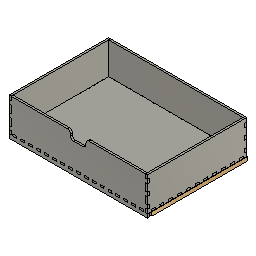
drawer (Autodesk Fusion 360 design; units mm, degrees)
Autodesk Fusion 360 part; units mm, degrees
sketch "Drawer base geometry" plane through (0, 0, 0) normal (0, 0, 1) x (1, 0, 0)
  line L0 (0, 0) -> (362, 0)
  line L1 (362, 0) -> (362, 260)
  line L2 (362, 260) -> (0, 260)
  line L3 (0, 260) -> (0, 0)
  line L4 (1, 0) -> (361, 0)
  line L5 (361, 0) -> (361, 259)
  line L6 (361, 259) -> (1, 259)
  line L7 (1, 259) -> (1, 0)
  line L8 (6, 5) -> (356, 5)
  line L9 (356, 5) -> (356, 254)
  line L10 (356, 254) -> (6, 254)
  line L11 (6, 254) -> (6, 5)
  point P0 (1, 259)
  dimension "d14" = 362
  dimension "d15" = 260
  dimension "d16" = 1
  dimension "d17" = 1
  dimension "d18" = 1
  dimension "d21" = 5
  dimension "d22" = 5
  dimension "d23" = 5
  dimension "d24" = 5
  constraint horizontal L0
  constraint vertical L1
  constraint horizontal L2
  constraint vertical L3
  constraint coincident L0.start L3.end
  constraint horizontal L4
  constraint vertical L5
  constraint horizontal L6
  constraint vertical L7
  constraint horizontal L8
  constraint vertical L9
  constraint horizontal L10
  constraint vertical L11
  constraint collinear L0 L4
  constraint coincident P0 L6.end
  measures "d14" distance of L0.start L0.end
  measures "d15" distance of L0.start L2.end
  measures "d16" distance of L3 L7
  measures "d17" distance of L1 L5
  measures "d18" distance of L2 L6
  measures "d21" distance of L6 L10
  measures "d22" distance of L0 L8
  measures "d23" distance of L5 L9
  measures "d24" distance of L7 L11
ref_plane "WorkPlane1" through (6, 129.5, 0) normal (-1, 0, 0) x (0, -1, 0)
ref_plane "WorkPlane2" through (181, 254, 0) normal (0, 1, 0) x (-1, 0, 0)
sketch "Tabs side" plane through (6, 99.5, 0) normal (-1, 0, 0) x (0, 1, 0)
  line L0 (-99.5, 0) -> (159.5, 0)
  line L1 (159.5, 0) -> (159.5, -88)
  line L2 (159.5, -88) -> (-99.5, -88)
  line L3 (-99.5, -88) -> (-99.5, 0)
  line L4 (-89.5, -5) -> (-79.5, -5)
  line L5 (-79.5, -5) -> (-79.5, 0)
  line L6 (-79.5, 0) -> (-89.5, 0)
  line L7 (-89.5, 0) -> (-89.5, -5)
  line L8 (-99.5, -44) -> (159.5, -44) construction
  line L9 (30, -88) -> (30, 0) construction
  line L10 (-99.5, -10) -> (-94.5, -10)
  line L11 (-94.5, -10) -> (-94.5, -20)
  line L12 (-94.5, -20) -> (-99.5, -20)
  line L13 (-99.5, -20) -> (-99.5, -10)
  point P0 (-99.5, 0)
  dimension "d27" = 259
  dimension "d28" = 88
  dimension "d36" = 10
  dimension "d37" = 10
  dimension "d38" = 5
  dimension "d39" = 10
  dimension "d40" = 5
  dimension "d41" = 10
  constraint horizontal L0
  constraint vertical L1
  constraint horizontal L2
  constraint vertical L3
  constraint coincident P0 L0.start
  constraint horizontal L4
  constraint vertical L5
  constraint horizontal L6
  constraint vertical L7
  constraint midpoint L3 L8.start
  constraint midpoint L1 L8.end
  constraint midpoint L2 L9.start
  constraint coincident L0 L9.end
  constraint perpendicular L0 L9
  constraint collinear L0 L6
  constraint horizontal L10
  constraint vertical L11
  constraint horizontal L12
  constraint vertical L13
  constraint collinear L3 L13
  measures "d27" distance of L1.end L2.end
  measures "d28" distance of P0 L2.end
  measures "d36" distance of L3 L7
  measures "d37" distance of L4.start L4.end
  measures "d38" distance of L0 L4
  measures "d39" distance of L0 L10
  measures "d40" distance of L3 L11
  measures "d41" distance of L10 L12
extrude "Extrude1" add sketch "Tabs side" along normal blind 5 contours L0 L1 L2 L3 L4 L5 L7 L10 L11 L12 makes body 1
ref_plane "WorkPlane3" through (3.5, 139.5, 44) normal (0, 0, -1) x (0, -1, 0)
ref_plane "WorkPlane4" through (3.5, 129.5, 54) normal (0, -1, 0) x (0, 0, 1)
mirror "Mirror2" about plane through (3.5, 129.5, 54) normal (0, -1, 0) of 3 faces at (4.3333, 5, 13.3333) (4.3333, 3.3333, 20) (4.3333, 1.6667, 10) on bodies 1
pattern_linear "R-Pattern2" count 3 spacing 29 along (0, 0, 1) of 6 faces at (4.3333, 5, 13.3333) (4.3333, 3.3333, 20) (4.3333, 1.6667, 10) (4.3333, 257.3333, 10) (4.3333, 254, 13.3333) (4.3333, 255.6667, 20) on bodies 1
pattern_linear "R-Pattern3" count 11 spacing 22.9 along (0, 1, 0) of 3 faces at (4.3333, 10, 1.6667) (4.3333, 13.3333, 5) (4.3333, 20, 3.3333) on bodies 1
sketch "Tab rear" plane through (125, 254, 0) normal (0, 1, 0) x (1, 0, 0)
  line L0 (-124, -88) -> (-124, 0)
  line L1 (-114, 0) -> (-104, 0)
  line L2 (-104, 0) -> (-104, -5)
  line L3 (-104, -5) -> (-114, -5)
  line L4 (-114, -5) -> (-114, 0)
  line L5 (-124, 0) -> (236, 0)
  line L6 (236, 0) -> (236, -88)
  line L7 (236, -88) -> (-124, -88)
  point P0 (-124, 0)
  dimension "d61" = 10
  dimension "d63" = 10
  dimension "d100" = 360
  dimension "d101" = 88
  dimension "d102" = 5
  constraint vertical L0
  constraint coincident P0 L0.end
  constraint horizontal L1
  constraint vertical L2
  constraint horizontal L3
  constraint vertical L4
  constraint perpendicular L4 L5
  constraint perpendicular L5 L6
  constraint parallel L5 L7
  constraint collinear L1 L5
  measures "d61" distance of L0 L4
  measures "d63" distance of L2 L4
  measures "d100" distance of P0 L5.end
  measures "d101" distance of L5 L7
  measures "d102" distance of L3 L5
extrude "Extrude2" add sketch "Tab rear" along normal blind 5 separate body contours L0 L2 L3 L4 L5 L6 L7 makes body 2
pattern_linear "R-Pattern4" count 17 spacing 20.625 along (1, 0, 0) of 3 faces at (11, 255.6667, 3.3333) (17.6667, 255.6667, 5) (21, 255.6667, 1.6667) on bodies 2
ref_plane "WorkPlane5" through (181, 0, 0) normal (1, 0, 0) x (0, 1, 0)
mirror "Mirror3" about plane through (181, 0, 0) normal (1, 0, 0) of bodies 1 makes body 3
combine "Combine1" operation cut target body 2 tool bodies 1 3 keep tools
ref_plane "WorkPlane6" through (0, 129.5, 0) normal (0, 1, 0) x (0, 0, 1)
mirror "Mirror4" about plane through (0, 129.5, 0) normal (0, 1, 0) of bodies 2 makes body 4
extrude "Extrude3" add sketch "Drawer base geometry" along normal blind 5 separate body contours L0 L4 L5 L6 L7 | L8 L9 L10 L11 makes body 5
combine "Combine2" operation cut target body 5 tool bodies 2 1 3 4 keep tools
sketch "Front lip" plane through (0, 0, 0) normal (0, 1, 0) x (1, 0, 0)
  line L0 (1, 0) -> (361, 0)
  line L1 (361, 0) -> (361, 9.5)
  line L2 (361, 9.5) -> (1, 9.5)
  line L3 (1, 9.5) -> (1, 0)
  point P0 (1, 0)
  dimension "d78" = 360
  dimension "d80" = 9.5
  constraint horizontal L0
  constraint vertical L1
  constraint horizontal L2
  constraint vertical L3
  constraint coincident P0 L0.start
  measures "d78" distance of L1.end L2.end
  measures "d80" distance of L0 L2
extrude "Extrude4" add sketch "Front lip" along normal blind 5 separate body makes body 6
combine "Combine3" operation add target body 4 tool bodies 6
sketch "Rail" plane through (0, 0, 0) normal (1, 0, 0) x (0, 1, 0)
  line L0 (259, 0) -> (11, 0)
  line L1 (11, 0) -> (11, -10)
  line L2 (11, -10) -> (259, -10)
  line L3 (259, -10) -> (259, 0)
  point P0 (259, 0)
  dimension "d83" = 10
  dimension "d84" = 248
  constraint horizontal L0
  constraint vertical L1
  constraint horizontal L2
  constraint vertical L3
  constraint coincident P0 L0.start
  measures "d83" distance of L0.end L1.end
  measures "d84" distance of L1.end L2.end
extrude "Extrude5" add sketch "Rail" along normal blind 10 separate body makes body 7
mirror "Mirror5" about plane through (181, 0, 0) normal (1, 0, 0) of bodies 7 makes body 8
sketch "Front hole" plane through (0, 0, 0) normal (0, -1, 0) x (1, 0, 0)
  line L0 (356, 0) -> (356, 10)
  line L1 (356, 10) -> (361, 10)
  line L2 (361, 10) -> (361, 20)
  line L3 (361, 20) -> (356, 20)
  line L4 (356, 20) -> (356, 39)
  line L5 (356, 39) -> (361, 39)
  line L6 (361, 39) -> (361, 49)
  line L7 (361, 49) -> (356, 49)
  line L8 (356, 49) -> (356, 68)
  line L9 (356, 68) -> (361, 68)
  line L10 (361, 68) -> (361, 78)
  line L11 (361, 78) -> (356, 78)
  line L12 (356, 78) -> (356, 88)
  line L13 (356, 88) -> (6, 88)
  line L14 (6, 88) -> (6, 78)
  line L15 (6, 78) -> (1, 78)
  line L16 (1, 78) -> (1, 68)
  line L17 (1, 68) -> (6, 68)
  line L18 (6, 68) -> (6, 49)
  line L19 (6, 49) -> (1, 49)
  line L20 (1, 49) -> (1, 39)
  line L21 (1, 39) -> (6, 39)
  line L22 (6, 39) -> (6, 20)
  line L23 (6, 20) -> (1, 20)
  line L24 (1, 20) -> (1, 10)
  line L25 (1, 10) -> (6, 10)
  line L26 (6, 10) -> (6, 0)
  line L27 (6, 0) -> (1, 0)
  line L28 (1, 0) -> (1, -9.5)
  line L29 (1, -9.5) -> (361, -9.5)
  line L30 (361, -9.5) -> (361, 0)
  line L31 (361, 0) -> (356, 0)
  line L32 (351, 0) -> (341, 0)
  line L33 (341, 0) -> (341, 5)
  line L34 (341, 5) -> (351, 5)
  line L35 (351, 5) -> (351, 0)
  line L36 (11, 0) -> (11, 5)
  line L37 (11, 5) -> (21, 5)
  line L38 (21, 5) -> (21, 0)
  line L39 (21, 0) -> (11, 0)
  line L40 (31.625, 0) -> (31.625, 5)
  line L41 (31.625, 5) -> (41.625, 5)
  line L42 (41.625, 5) -> (41.625, 0)
  line L43 (41.625, 0) -> (31.625, 0)
  line L44 (52.25, 0) -> (52.25, 5)
  line L45 (52.25, 5) -> (62.25, 5)
  line L46 (62.25, 5) -> (62.25, 0)
  line L47 (62.25, 0) -> (52.25, 0)
  line L48 (72.875, 0) -> (72.875, 5)
  line L49 (72.875, 5) -> (82.875, 5)
  line L50 (82.875, 5) -> (82.875, 0)
  line L51 (82.875, 0) -> (72.875, 0)
  line L52 (93.5, 0) -> (93.5, 5)
  line L53 (93.5, 5) -> (103.5, 5)
  line L54 (103.5, 5) -> (103.5, 0)
  line L55 (103.5, 0) -> (93.5, 0)
  line L56 (114.125, 0) -> (114.125, 5)
  line L57 (114.125, 5) -> (124.125, 5)
  line L58 (124.125, 5) -> (124.125, 0)
  line L59 (124.125, 0) -> (114.125, 0)
  line L60 (134.75, 0) -> (134.75, 5)
  line L61 (134.75, 5) -> (144.75, 5)
  line L62 (144.75, 5) -> (144.75, 0)
  line L63 (144.75, 0) -> (134.75, 0)
  line L64 (155.375, 0) -> (155.375, 5)
  line L65 (155.375, 5) -> (165.375, 5)
  line L66 (165.375, 5) -> (165.375, 0)
  line L67 (165.375, 0) -> (155.375, 0)
  line L68 (176, 0) -> (176, 5)
  line L69 (176, 5) -> (186, 5)
  line L70 (186, 5) -> (186, 0)
  line L71 (186, 0) -> (176, 0)
  line L72 (196.625, 0) -> (196.625, 5)
  line L73 (196.625, 5) -> (206.625, 5)
  line L74 (206.625, 5) -> (206.625, 0)
  line L75 (206.625, 0) -> (196.625, 0)
  line L76 (217.25, 0) -> (217.25, 5)
  line L77 (217.25, 5) -> (227.25, 5)
  line L78 (227.25, 5) -> (227.25, 0)
  line L79 (227.25, 0) -> (217.25, 0)
  line L80 (237.875, 0) -> (237.875, 5)
  line L81 (237.875, 5) -> (247.875, 5)
  line L82 (247.875, 5) -> (247.875, 0)
  line L83 (247.875, 0) -> (237.875, 0)
  line L84 (258.5, 0) -> (258.5, 5)
  line L85 (258.5, 5) -> (268.5, 5)
  line L86 (268.5, 5) -> (268.5, 0)
  line L87 (268.5, 0) -> (258.5, 0)
  line L88 (279.125, 0) -> (279.125, 5)
  line L89 (279.125, 5) -> (289.125, 5)
  line L90 (289.125, 5) -> (289.125, 0)
  line L91 (289.125, 0) -> (279.125, 0)
  line L92 (299.75, 0) -> (299.75, 5)
  line L93 (299.75, 5) -> (309.75, 5)
  line L94 (309.75, 5) -> (309.75, 0)
  line L95 (309.75, 0) -> (299.75, 0)
  line L96 (330.375, 0) -> (320.375, 0)
  line L97 (320.375, 0) -> (320.375, 5)
  line L98 (320.375, 5) -> (330.375, 5)
  line L99 (330.375, 5) -> (330.375, 0)
  line L100 (181, 88) -> (181, 0) construction
  line L101 (161, 88) -> (201, 88)
  line L102 (201, 88) -> (201, 68)
  line L103 (201, 68) -> (161, 68)
  line L104 (161, 68) -> (161, 88)
  point P0 (181, 88)
  point P1 (181, 88)
  dimension "d103" = 20
  dimension "d104" = 40
  constraint midpoint L13 P1
  constraint coincident P1 P0
  constraint midpoint L71 L100.end
  constraint horizontal L101
  constraint vertical L102
  constraint horizontal L103
  constraint vertical L104
  constraint midpoint L101 P1
  measures "d103" distance of L101.end L102.end
  measures "d104" distance of L101.start L101.end
extrude "Extrude8" cut sketch "Front hole" against normal up to surface (5 mm away) contours L13 L101 L102 L103 L104 bodies 4
fillet "Fillet1" radius 8 4 edges at (161, 2.5, 88) (161, 2.5, 68) (201, 2.5, 88) (201, 2.5, 68) on bodies 4
equation "shelf_depth = 260 mm" comment "Depth of enclosing shelf"
equation "shelf_width = 362 mm" comment "Width of enclosing shelf"
equation "shelf_height = 300 mm" comment "Height of enclosing shelf"
equation "clearance_side = 1 mm" comment "How much spacce room the drawer has on each side"
equation "clearance_back = 1 mm" comment "How much space the drawer has towards the back of the shelf"
equation "clearance_top = 2 mm" comment "How much space the top of the drawer has"
equation "drawer_width = shelf_width - ( 2 * clearance_side )" comment "Drawer width"
equation "drawer_depth = shelf_depth - clearance_back" comment "Drawer depth"
equation "num_drawers = 3 mm" comment "Number of drawers we want in the shelf"
equation "rail_height = 10 mm" comment "Hight of the rail the drawer rests on"
equation "rail_width = 10 mm" comment "Width of the rail the drawer rests on"
equation "rail_depth = shelf_depth - ( 2 * clearance_back ) - ( 2 * material_thickness )" comment "Depth of the rail the drawer rests on"
equation "drawer_height = ( ( shelf_height / num_drawers ) * 1 mm ) - rail_height - clearance_top" comment "Height of the drawer"
equation "d14 = shelf_width"
equation "d15 = shelf_depth"
equation "d16 = clearance_side"
equation "d17 = clearance_side"
equation "d18 = clearance_back"
equation "material_thickness = 5 mm" comment "Thickness of the drawer material"
equation "d21 = material_thickness"
equation "d22 = material_thickness"
equation "d23 = material_thickness"
equation "d24 = material_thickness"
equation "d27 = drawer_depth"
equation "d28 = drawer_height"
equation "tab_size = 2 * material_thickness" comment "Width of the tabs"
equation "tab_num_depth = floor(( ( drawer_depth - ( 4 * material_thickness ) ) / tab_size ) / 2)" comment "Number of tabs along the side panels"
equation "tab_num_height = floor(( ( drawer_height - ( 4 * material_thickness ) ) / tab_size ) / 2)" comment "Number of tabs vertically"
equation "d36 = 2 * material_thickness"
equation "d37 = tab_size"
equation "d38 = material_thickness"
equation "d39 = 2 * material_thickness"
equation "d40 = material_thickness"
equation "d41 = tab_size"
equation "d42 = material_thickness"
equation "d50 = tab_num_height"
equation "d52 = -drawer_height + ( 4 * material_thickness ) + tab_size"
equation "d54 = tab_num_depth"
equation "d56 = drawer_depth - ( 4 * material_thickness ) - tab_size"
equation "d61 = 2 * material_thickness"
equation "d63 = tab_size"
equation "d64 = material_thickness"
equation "d66 = tab_num_width"
equation "d68 = -drawer_width + ( 4 * material_thickness ) + tab_size"
equation "tab_num_width = floor(( ( drawer_width - ( 4 * material_thickness ) ) / tab_size ) / 2)" comment "Number of tabs across"
equation "d72 = ( drawer_width / 2 ) + clearance_side"
equation "d74 = drawer_depth / 2"
equation "d76 = material_thickness"
equation "d78 = drawer_width"
equation "bottom_lip_height = rail_height - clearance_bottom_lip" comment "How far below the bottom of the drawer the bottom lip protrudes"
equation "d80 = bottom_lip_height"
equation "d81 = material_thickness"
equation "d83 = rail_height"
equation "d84 = rail_depth"
equation "d85 = rail_width"
equation "clearance_bottom_lip = 0.5 mm" comment "clearance of the bottom lip"
equation "d100 = drawer_width"
equation "d101 = drawer_height"
equation "d102 = material_thickness"
equation "d103 = front_hole_height"
equation "d104 = front_hole_width"
equation "front_hole_width = 40 mm"
equation "front_hole_height = 20 mm"
equation "front_hole_corner_radius = 8 mm"
equation "d110 = front_hole_corner_radius"
named bodies: "Left side", "Back", "Right side", "Bottom", "Left rail", "Right rail", "Front"
